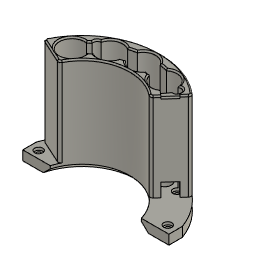
18650UPSBasement v3 (Autodesk Fusion 360 design; units mm, degrees)
Autodesk Fusion 360 part; units mm, degrees
sketch "Sketch1" plane through (0, 0, 0) normal (0, 0, 1) x (1, 0, 0) in component "BasementBase v4"
  circle A0 centre (0, 50) radius 1.6
  circle A1 centre (0, 0) radius 40
  line L0 (0, 0) -> (0, 50) construction
  circle A2 centre (-47.5528, 15.4509) radius 1.6
  line L1 (53.8012, 10.0063) -> (53.8006, 20.0063)
  arc A3 (53.8006, 20.0063) -> (-53.803, 20) centre (0, 0) ccw
  circle A4 centre (47.5528, 15.4509) radius 1.6
  circle A5 centre (-29.3893, 40.4508) radius 1.6
  circle A6 centre (29.3893, 40.4508) radius 1.6
  line L2 (-53.803, 20) -> (-53.8024, 10)
  line L3 (-53.8024, 10) -> (53.8012, 10.0063)
  circle A7 centre (0, 0) radius 50 construction
  line L4 (-53.8024, 10) -> (-53.8018, 0) construction
  line L5 (-53.8018, 0) -> (0, 0) construction
  circle A8 centre (0, 0) radius 25
  circle A9 centre (-47.5528, 15.4509) radius 3
  circle A10 centre (-29.3893, 40.4508) radius 3
  circle A11 centre (0, 50) radius 3
  circle A12 centre (29.3893, 40.4508) radius 3
  circle A13 centre (47.5528, 15.4509) radius 3
  dimension "d268" = 3.2
  dimension "d13" = 80
  dimension "d14" = 57.4
  dimension "d16" = 30.9017
  dimension "d17" = 30.9017
  dimension "d18" = 30.9017
  dimension "d19" = 30.9017
  dimension "d20" = 10
  dimension "d21" = 10
  dimension "d22" = 100
  dimension "d23" = 3.2
  dimension "d24" = 3.2
  dimension "d25" = 3.2
  dimension "d26" = 3.2
  dimension "d32" = 50
  dimension "d33" = 6
  dimension "d34" = 6
  dimension "d35" = 6
  dimension "d36" = 6
  dimension "d37" = 6
  constraint coincident A1.centre L0.start
  constraint coincident A0.centre L0.end
  constraint coincident L2 L3.start
  constraint coincident L1 L3.end
  constraint perpendicular L1 L3
  constraint coincident A0.centre A7
  constraint vertical L0
  constraint perpendicular L2 L3
  constraint equal L1 L2
  constraint coincident L1.start L3.end
  constraint coincident A2.centre A7
  constraint coincident A5.centre A7
  constraint coincident A6.centre A7
  constraint coincident A4.centre A7
  constraint perpendicular L3 L4
  constraint perpendicular L0 L5
  constraint concentric A4 A13
  constraint coincident A2.centre A9.centre
  constraint coincident A5.centre A10.centre
  constraint coincident A6.centre A12.centre
  measures "d268" diameter of A0
  measures "d13" diameter of A1
  measures "d14" radius of A3
  measures "d16" distance of A5.centre A0.centre
  measures "d17" distance of A5.centre A2.centre
  measures "d18" distance of A0.centre A6.centre
  measures "d19" distance of A4.centre A6.centre
  measures "d20" distance of A3.end L2.end
  measures "d21" distance of L2.end L4.end
  measures "d22" diameter of A7
  measures "d23" diameter of A2
  measures "d24" diameter of A5
  measures "d25" diameter of A6
  measures "d26" diameter of A4
  measures "d32" diameter of A8
  measures "d33" diameter of A9
  measures "d34" diameter of A10
  measures "d35" diameter of A11
  measures "d36" diameter of A12
  measures "d37" diameter of A13
extrude "Extrude1" add sketch "Sketch1" against normal blind 5 contours A1 L1 A3 L2 L3 | A9 | A10 | A11 | A12 | A13 in component "BasementBase v4"
extrude "Extrude2" add sketch "Sketch1" along normal blind 2 contours A1 L3 A8 | A1 L1 A3 L2 L3 picked at (-31.3201, 15.4348) in component "BasementBase v4"
chamfer "Chamfer1" distance 5 angle 45 1 edges at (-0.0024, 40, 0) in component "BasementBase v4"
sketch "Sketch1 (2)" plane through (0, 0, 2) normal (0, 0, 1) x (-1, 0, 0)
  circle A0 centre (47.5528, -15.4509) radius 3
  circle A1 centre (-29.3893, -40.4508) radius 3
  circle A2 centre (0, -50) radius 3
  circle A3 centre (29.3893, -40.4508) radius 3
  circle A4 centre (-47.5528, -15.4509) radius 3
  line L0 (-22.9109, -10.0045) -> (-53.8012, -10.0063)
  line L1 (-53.8012, -10.0063) -> (-53.8006, -20.0063)
  arc A5 (-53.8006, -20.0063) -> (53.803, -20) centre (0, 0) ccw
  line L2 (53.803, -20) -> (53.8024, -10)
  line L3 (53.8024, -10) -> (22.9121, -10.0018)
  arc A6 (-22.9109, -10.0045) -> (22.9121, -10.0018) centre (0, 0) ccw
  circle A7 centre (36.1067, -28.501) radius 9.25
  circle A8 centre (20.5985, -41.1303) radius 9.25
  circle A9 centre (1.1965, -45.9844) radius 9.25
  circle A10 centre (-18.4316, -42.1459) radius 9.25
  circle A11 centre (0, 0) radius 46
  circle A12 centre (0, 0) radius 57.4
  circle A13 centre (0, 0) radius 35
  line L4 (0, 0) -> (-34.9082, -45.5651)
  line L5 (0, 0) -> (-38.7467, -42.3492)
  line L6 (0, 0) -> (52.2522, -23.7585)
  circle A14 centre (0, 0) radius 51
  circle A15 centre (0, 0) radius 41
  circle A16 centre (36.1067, -28.501) radius 5
  circle A17 centre (20.5985, -41.1303) radius 5
  circle A18 centre (1.1965, -45.9844) radius 5
  circle A19 centre (-18.4316, -42.1459) radius 5
  dimension "d1" = 18.5
  dimension "d2" = 18.5
  dimension "d3" = 18.5
  dimension "d4" = 18.5
  dimension "d5" = 92
  dimension "d6" = 20
  dimension "d7" = 20
  dimension "d8" = 20
  dimension "d9" = 70
  dimension "d10" = 18.5
  dimension "d11" = 11
  dimension "d12" = 11
  dimension "d41" = 102
  dimension "d42" = 82
  dimension "d43" = 5
  dimension "d51" = 10
  dimension "d52" = 10
  dimension "d53" = 10
  dimension "d54" = 10
  constraint coincident A5.centre A6.centre
  constraint coincident A7.centre A11
  constraint coincident A8.centre A11
  constraint coincident A9.centre A11
  constraint coincident A10.centre A11
  constraint concentric A11 A12
  constraint coincident A12 L4.end
  constraint coincident A5 L4.end
  constraint coincident A12 L5.end
  constraint coincident A12 L6.end
  constraint concentric A12 A15
  constraint concentric A7 A16
  constraint concentric A8 A17
  constraint concentric A9 A18
  constraint concentric A10 A19
  measures "d1" diameter of A7
  measures "d2" diameter of A8
  measures "d3" diameter of A9
  measures "d4" diameter of A10
  measures "d5" diameter of A11
  measures "d6" distance of A7.centre A8.centre
  measures "d7" distance of A8.centre A9.centre
  measures "d8" distance of A9.centre A10.centre
  measures "d9" diameter of A13
  measures "d10" distance of L3 A7.centre
  measures "d11" distance of A10.centre L4
  measures "d12" distance of A7.centre L6
  measures "d41" diameter of A14
  measures "d42" diameter of A15
  measures "d43" angle of L4 L5
  measures "d51" diameter of A16
  measures "d52" diameter of A17
  measures "d53" diameter of A18
  measures "d54" diameter of A19
extrude "Extrude3" cut sketch "Sketch1 (2)" against normal blind 7 contours A11 A16 | L3 A6 A13 L6 | A11 A16 | A6 A13 L4 L6 | A6 A13 L4 L5 | L0 A6 A13 L5 | A11 A17 | A11 A19 | A11 A17 | A11 A19 | A2 A14 | A2 A14 A18 | A11 A18 | A2 A11 A18 | A2 A14 A18 | A2 A18 in component "BasementBase v4"
extrude "Extrude4" add sketch "Sketch1 (2)" along normal blind 65 contours A7 A11 L6 A14 | A1 A3 A5 A7 A8 A9 A10 A12 L4 L6 A14 | A7 A11 L6 A15 | A7 A8 A9 A10 A13 L4 L6 A15 | A1 A5 A12 L4 L5 A14 | A13 L4 L5 A15 in component "BasementBase v4"
extrude "Extrude5" add sketch "Sketch1 (2)" along normal blind 54 from surface at 10 contours A11 L4 L5 A15 | A1 A11 L4 L5 A14 in component "BasementBase v4"
fillet "Fillet1" radius 2 4 edges at (-52.2522, 23.7585, 34.5) (-31.8611, 14.4869, 34.5) (23.626, 25.8227, 34.5) (38.7467, 42.3492, 34.5) in component "BasementBase v4"
fillet "Fillet2" radius 1 10 edges at (23.6067, 26.6135, 67) (35.8994, 39.2372, 67) (26.3079, 28.7539, 67) (31.0513, 33.9384, 66) (37.8927, 42.3219, 67) (-11.4893, 56.2384, 67) (-51.456, 24.0683, 67) (-42.0156, 19.1041, 67) (-32.1535, 15.2219, 67) (-7.0056, 34.2917, 67) in component "BasementBase v4"
fillet "Fillet3" radius 1 15 edges at (-42.4323, 21.7521, 67) (-33.3608, 38.5754, 67) (-31.8659, 42.1439, 67) (-23.7695, 49.8198, 67) (-12.3781, 49.4751, 67) (-1.4372, 55.2313, 67) (9.7883, 50.0519, 67) (22.1173, 50.6299, 67) (31.1682, 42.8665, 67) (14.7253, 33.6709, 67) (7.869, 40.2378, 67) (-0.9559, 36.7376, 67) (-16.4564, 32.8595, 67) (-9.951, 39.7741, 67) (-25.89, 31.7917, 67) in component "BasementBase v4"
component "BasementBase v4" placed x (1, 0, 0) y (0, 1, 0) z (0, 0, 1) at (0, 0, 0)
